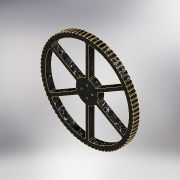
# Autodesk Inventor part: Llana
Saved by Autodesk Inventor 2021 (Build 250183000, 183)
## iProperties
Created: 2024-04-09
Part Number: Llana
Material: PLA
Document SubType Name: Modeling
Designer: Martin
Density: 1.27 g/cm^3
Appearance: PLA
Mass: 23.2917 g
Surface Area: 110.693 cm^2
Volume: 18.3399 cm^3
Author: Martin
Autodesk Inventor part; units mm, degrees
ref_plane "YZ Plane" through (0, 0, 0) normal (1, 0, 0) x (0, 1, 0)
ref_plane "XZ Plane" through (0, 0, 0) normal (0, 1, 0) x (-1, 0, 0)
ref_plane "XY Plane" through (0, 0, 0) normal (0, 0, 1) x (1, 0, 0)
sketch "Sketch1" plane through (0, 0, 0) normal (0, 0, 1) x (1, 0, 0)
  circle A0 centre (0, 0) radius 75
  line L0 (-2.5, 19.056713) -> (-2.5, 65.921316)
  line L1 (2.5, 19.056713) -> (2.5, 65.937337)
  line L2 (0, -106.489337) -> (0, 113.936021)
  arc A1 (-2.5, 65.921316) -> (-4.189356, 67.409316) centre (-4, 65.921316) ccw
  arc A2 (4.330984, 67.400365) -> (2.5, 65.937337) centre (4, 65.937337) ccw
  arc A3 (-3.96867, 17.55704) -> (-2.5, 19.056713) centre (-4, 19.056713) ccw
  arc A4 (2.5, 19.056713) -> (3.96867, 17.55704) centre (4, 19.056713) ccw
  arc A5 (-15.253598, 11.69342) -> (-13.220508, 12.215489) centre (-14.503598, 12.992458) ccw
  arc A6 (-17.189178, 5.341551) -> (-17.753598, 7.363293) centre (-18.503598, 6.064255) ccw
  line L3 (-17.753598, 7.363293) -> (-58.339534, 30.795594)
  line L4 (-15.253598, 11.69342) -> (-55.853409, 35.133732)
  arc A7 (-56.204936, 37.450925) -> (-55.853409, 35.133732) centre (-55.103409, 36.43277) ccw
  arc A8 (-58.339534, 30.795594) -> (-60.472858, 30.076569) centre (-59.089534, 29.496556) ccw
  arc A9 (-17.753598, -7.363293) -> (-17.189178, -5.341551) centre (-18.503598, -6.064255) ccw
  arc A10 (-13.220508, -12.215489) -> (-15.253598, -11.69342) centre (-14.503598, -12.992458) ccw
  line L5 (-15.253598, -11.69342) -> (-55.839534, -35.125721)
  line L6 (-17.753598, -7.363293) -> (-58.353409, -30.803605)
  arc A11 (-60.53592, -29.94944) -> (-58.353409, -30.803605) centre (-59.103409, -29.504567) ccw
  arc A12 (-55.839534, -35.125721) -> (-56.283502, -37.332747) centre (-55.089534, -36.42476) ccw
  arc A13 (-2.5, -19.056713) -> (-3.96867, -17.55704) centre (-4, -19.056713) ccw
  arc A14 (3.96867, -17.55704) -> (2.5, -19.056713) centre (4, -19.056713) ccw
  line L7 (2.5, -19.056713) -> (2.5, -65.921316)
  line L8 (-2.5, -19.056713) -> (-2.5, -65.937337)
  arc A15 (-4.330984, -67.400365) -> (-2.5, -65.937337) centre (-4, -65.937337) ccw
  arc A16 (2.5, -65.921316) -> (4.189356, -67.409316) centre (4, -65.921316) ccw
  arc A17 (15.253598, -11.69342) -> (13.220508, -12.215489) centre (14.503598, -12.992458) ccw
  arc A18 (17.189178, -5.341551) -> (17.753598, -7.363293) centre (18.503598, -6.064255) ccw
  line L9 (17.753598, -7.363293) -> (58.339534, -30.795594)
  line L10 (15.253598, -11.69342) -> (55.853409, -35.133732)
  arc A19 (56.204936, -37.450925) -> (55.853409, -35.133732) centre (55.103409, -36.43277) ccw
  arc A20 (58.339534, -30.795594) -> (60.472858, -30.076569) centre (59.089534, -29.496556) ccw
  arc A21 (-4.189356, 67.409316) -> (-56.204936, 37.450925) centre (0, 0) ccw
  arc A22 (-3.96867, 17.55704) -> (-13.220508, 12.215489) centre (0, 0) ccw
  arc A23 (-17.189178, 5.341551) -> (-17.189178, -5.341551) centre (0, 0) ccw
  arc A24 (-60.472858, 30.076569) -> (-60.53592, -29.94944) centre (0, 0) ccw
  arc A25 (-56.283502, -37.332747) -> (-4.330984, -67.400365) centre (0, 0) ccw
  arc A26 (-13.220508, -12.215489) -> (-3.96867, -17.55704) centre (0, 0) ccw
  arc A27 (3.96867, -17.55704) -> (13.220508, -12.215489) centre (0, 0) ccw
  arc A28 (17.189178, -5.341551) -> (3.96867, 17.55704) centre (0, 0) ccw
  arc A29 (4.189356, -67.409316) -> (56.204936, -37.450925) centre (0, 0) ccw
  arc A30 (60.472858, -30.076569) -> (4.330984, 67.400365) centre (0, 0) ccw
  arc A31 (17.753598, 7.363293) -> (17.189178, 5.341551) centre (18.503598, 6.064255) ccw
  arc A32 (13.220508, 12.215489) -> (15.253598, 11.69342) centre (14.503598, 12.992458) ccw
  line L11 (15.253598, 11.69342) -> (55.839534, 35.125721)
  line L12 (17.753598, 7.363293) -> (58.353409, 30.803605)
  arc A33 (60.53592, 29.94944) -> (58.353409, 30.803605) centre (59.103409, 29.504567) ccw
  arc A34 (55.839534, 35.125721) -> (56.283502, 37.332747) centre (55.089534, 36.42476) ccw
  point P0 (13.220508, 12.215489)
  point P1 (17.189178, 5.341551)
  point P2 (60.319935, 30.3821)
  point P3 (56.392579, 37.167777)
  point P4 (13.590699, 11.802241)
  point P5 (17.01639, 5.86877)
  dimension "d0" = 150
  dimension "d2" = 5
  dimension "d5" = 3
  dimension "d6" = 3
  dimension "d7" = 3
  dimension "d8" = 3
  dimension "d12" = 360
  dimension "d72" = 18
  dimension "d73" = 1.5
  constraints: 68 point on circle, 35 centre point, 24 end point, 4 tangent, 2 coincident, 1 parallel, 1 vertical, 110 other
  measures "d0" diameter of A0
  measures "d2" distance between parallel lines of L1 L0
  measures "d5" diameter of A1
  measures "d6" diameter of A2
  measures "d7" diameter of A3
  measures "d8" diameter of A4
  measures "d72" radius of A28
  measures "d73" radius of A13
extrude "Extrusion1" add sketch "Sketch1" along normal mid plane 10 contours A0 L2 | L2 A0 | A28 A32 | A34 A30 | A32 L11 A34 A30 A33 L12 A31 A28 | A28 A31 | A33 A30
ref_plane "Work Plane1" through (0, 75, 0) normal (0, 1, 0) x (-1, 0, 0)
sketch "Sketch3" plane through (0, 75, 0) normal (0, 1, 0) x (-1, 0, 0)
  line L0 (-75, -5) -> (75, -5) projected
  line L1 (0.75, 5) -> (-0.75, 5)
  line L2 (-0.75, 5) -> (-0.75, -5)
  line L3 (-0.75, -5) -> (0.75, -5)
  line L4 (0.75, -5) -> (0.75, 5)
  line L5 (0.75, 5) -> (-0.75, -5) construction
  line L6 (-0.75, 5) -> (0.75, -5) construction
  point P0 (0, 0)
  point P1 (0.75, -5)
  dimension "d57" = 1.5
  constraints: 12 end point, 2 midpoint, 2 parallel, 1 horizontal, 1 perpendicular, 1 point on line
  measures "d57" distance of L3.end L2.end
extrude "Extrusion4" cut sketch "Sketch3" against normal blind 1
pattern_circular "Circular Pattern2" count 80 over 360 about axis through (0, 0, -10) along (0, 0, 1) of "Extrusion4"
sketch "Sketch4" plane through (0, 0, 5) normal (0, 0, 1) x (1, 0, 0)
  circle A0 centre (0, 0) radius 11
  circle A1 centre (0, 0) radius 10
  circle A2 centre (-8.75, 0) radius 1.25
  circle A3 centre (0, -8.75) radius 1.25
  circle A4 centre (8.75, 0) radius 1.25
  circle A5 centre (0, 8.75) radius 1.25
  line L0 (-105, 0) -> (105, 0) projected
  dimension "d63" = 22
  dimension "d64" = 1
  dimension "d65" = 2.5
  dimension "d68" = 360
  constraints: 6 centre point, 1 coincident, 1 point on line, 1 tangent, 9 other
  measures "d63" diameter of A0
  measures "d64" radial gap between concentric circles of A0 A1
  measures "d65" diameter of A2
extrude "Extrusion5" cut sketch "Sketch4" against normal blind 5 contours A5 | L0 A4 | A3 | A4 L0 | L0 A2 | A2 L0
equation "\"d6\" = d5"
equation "\"d7\" = d5"
equation "\"d8\" = d9"
equation "\"d9\" = 3"
body "Solid1"
